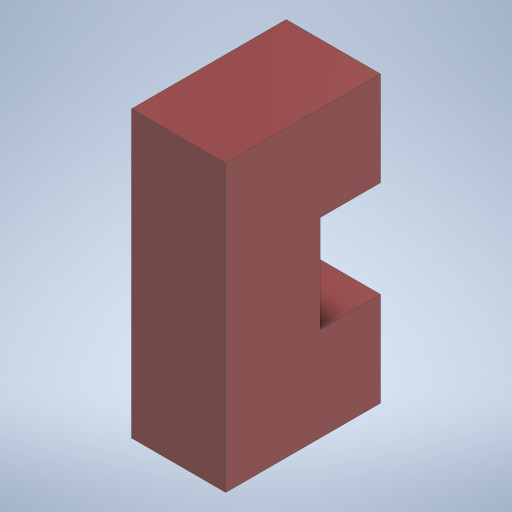
# Autodesk Inventor part: motor support
Saved by Autodesk Inventor 2024 (Build 280153000, 153)
## iProperties
Created: 2024-02-04
Part Number: motor support
Material: Generic
Document SubType Name: Modeling
Designer: RAHUL
Density: 1 g/cm^3
Appearance: Default
Author: RAHUL
Autodesk Inventor part; units mm, degrees
ref_plane "YZ Plane" through (0, 0, 0) normal (1, 0, 0) x (0, 1, 0)
ref_plane "XZ Plane" through (0, 0, 0) normal (0, 1, 0) x (-1, 0, 0)
ref_plane "XY Plane" through (0, 0, 0) normal (0, 0, 1) x (1, 0, 0)
sketch "Sketch1" plane through (0, 0, 0) normal (0, 0, 1) x (1, 0, 0)
  line L0 (0, 0) -> (39, 0)
  line L1 (39, 0) -> (39, 39)
  line L2 (39, 39) -> (0, 39)
  line L3 (0, 39) -> (0, 0)
  dimension "d0" = 39
  dimension "d1" = 39
  constraints: 8 end point, 2 parallel, 1 horizontal, 1 perpendicular
  measures "d0" distance of L2.end L1.end
  measures "d1" distance of L1.end L0.end
sketch "Sketch2" plane through (0, 0, 0) normal (1, 0, 0) x (0, 1, 0)
  line L0 (0, 0) -> (0, 25)
  line L1 (0, 25) -> (-40, 25)
  line L2 (-40, 25) -> (-40, 0)
  dimension "d2" = 25
  dimension "d3" = 40
  constraints: 6 end point, 1 horizontal, 1 perpendicular, 1 vertical
  measures "d2" distance of L0.start L0.end
  measures "d3" distance of L0.end L1.end
sweep "Sweep1" add profiles "Sketch1" path "Sketch2"
body "Solid1"
